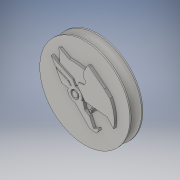
# Autodesk Inventor part: RTS Small Pharah Wheel
Saved by Autodesk Inventor 2016 (Build 200138000, 138)
## iProperties
Created: 2017-09-05
Part Number: RTS Small Pharah Wheel
Material: Generic
Document SubType Name: Modeling
Designer: Student
Density: 1 g/cm^3
Appearance: Default
Author: Student
Autodesk Inventor part; units mm, degrees
ref_plane "YZ Plane" through (0, 0, 0) normal (1, 0, 0) x (0, 1, 0)
ref_plane "XZ Plane" through (0, 0, 0) normal (0, 1, 0) x (-1, 0, 0)
ref_plane "XY Plane" through (0, 0, 0) normal (0, 0, 1) x (1, 0, 0)
sketch "Sketch1" plane through (0, 0, 0) normal (0, 0, 1) x (1, 0, 0)
  circle A0 centre (0, 0) radius 21.971
  dimension "d0" = 43.942
  constraints: 1 centre point, 1 coincident
  measures "d0" diameter of A0
extrude "Extrusion1" add sketch "Sketch1" along normal blind 6.35
sketch "Sketch3" plane through (0, 0, 0) normal (1, 0, 0) x (0, 1, 0)
  line L0 (21.971, 0) -> (21.971, 6.35) projected
  circle A0 centre (21.971, 3.175) radius 2.54
  line L1 (0, -1.27) -> (0, 7.62) projected
  point P0 (0, 0)
  dimension "d37" = 5.08
  constraints: 1 centre point, 1 midpoint
  measures "d37" diameter of A0
revolve "Revolution1" cut sketch "Sketch3" angle 360 about axis through (0, 0, -10) along (0, 0, 1)
sketch "Sketch4" plane through (0, 0, 0) normal (0, 0, -1) x (-1, 0, 0)
  line L0 (2.4384, -2.5883) -> (2.4384, 2.5883)
  line L1 (-2.4384, -2.5883) -> (-2.4384, 2.5883)
  arc A0 (2.4384, 2.5883) -> (-2.4384, 2.5883) centre (0, 0) ccw
  arc A1 (-2.4384, -2.5883) -> (2.4384, -2.5883) centre (0, 0) ccw
  dimension "d44" = 4.8768
  dimension "d45" = 3.556
  dimension "d46" = 5.1766
  dimension "d47" = 2.4384
  constraints: 4 end point, 4 point on circle, 2 centre point, 1 coincident, 1 parallel, 1 vertical
  measures "d44" distance between parallel lines of L1 L0
  measures "d45" radius of A0
  measures "d46" distance of L0.start L0.end
  measures "d47" distance from line of point (0, 0) L0
extrude "Extrusion3" cut sketch "Sketch4" against normal blind 5.2324
sketch "Sketch7" plane through (0, 0, 6.35) normal (0, 0, 1) x (1, 0, 0)
  line L0 (-16.6095, 17.2761) -> (16.9999, 17.2761) construction
  line L1 (16.9999, 17.2761) -> (16.9999, -16.3333) construction
  line L2 (16.9999, -16.3333) -> (-16.6095, -16.3333) construction
  line L3 (-16.6095, -16.3333) -> (-16.6095, 17.2761) construction
  line L4 (-11.6409, 13.9515) -> (-11.0896, 7.9216)
  line L5 (-10.846, 7.5655) -> (-4.1655, 4.5831)
  line L6 (-4.1655, 4.5831) -> (-3.2803, 2.7793)
  line L7 (-2.9643, 2.5005) -> (-2.215, 2.3615)
  arc A0 (-3.2803, 2.7793) -> (-2.9643, 2.5005) centre (-2.9521, 2.8328) ccw
  arc A1 (-11.0896, 7.9216) -> (-10.846, 7.5655) centre (-10.7308, 7.9057) ccw
  line L8 (-2.215, 2.3615) -> (-1.2053, 1.1357)
  circle A2 centre (-3.5155, -1.6738) radius 1.3912
  circle A3 centre (-3.5155, -1.6738) radius 1.9873
  arc A4 (-5.697, 1.0386) -> (-5.3458, 1.287) centre (-3.5155, -1.6738) ccw
  line L9 (-11.6409, 13.9515) -> (-10.9777, 13.9515)
  line L10 (-10.9777, 13.9515) -> (-6.6742, 11.6126)
  arc A5 (1.1675, 10.7462) -> (-6.6742, 11.6126) centre (-5.8633, -16.9682) ccw
  line L11 (1.1675, 10.7462) -> (2.608, 13.5351)
  arc A6 (3.3361, 13.55) -> (2.608, 13.5351) centre (2.9847, 12.9251) ccw
  line L12 (3.3361, 13.55) -> (10.8059, 7.7029)
  line L13 (10.8059, 7.7029) -> (13.5308, 5.0781)
  arc A7 (15.3657, -6.8873) -> (13.5308, 5.0781) centre (-3.032, -3.5852) ccw
  line L14 (15.3657, -6.8873) -> (12.1684, -3.357)
  line L15 (12.1684, -3.357) -> (7.5314, -2.8768)
  line L16 (7.5314, -2.8768) -> (7.0204, -3.2978)
  arc A8 (7.0204, -3.2978) -> (6.2865, -4.1165) centre (8.4411, -5.3095) ccw
  arc A9 (6.691, -2.8601) -> (6.2865, -4.1165) centre (9.098, -4.3284) ccw
  arc A10 (1.2675, -2.0364) -> (1.5721, -2.2799) centre (1.8757, -1.5881) ccw
  line L17 (1.2675, -2.0364) -> (-0.2802, -0.051)
  line L18 (-1.2053, 1.1357) -> (-0.2802, -0.051)
  line L19 (-15.1657, 8.8933) -> (-15.0771, 9.0065)
  line L20 (-15.0771, 9.0065) -> (-4.5214, 4.1672)
  line L21 (-4.5214, 4.1672) -> (-3.3907, 1.9212)
  line L22 (-6.652, 2.1979) -> (-5.6743, 1.0111)
  line L23 (-6.3027, 2.5826) -> (-5.3012, 1.2266)
  arc A11 (-5.6743, 1.0111) -> (-5.3012, 1.2266) centre (-5.5057, 1.15) ccw
  arc A12 (-6.652, 2.1979) -> (-7.0642, 2.431) centre (-7.2707, 1.5847) ccw
  arc A13 (-6.3027, 2.5826) -> (-6.6404, 2.7727) centre (-6.6833, 2.3015) ccw
  line L24 (-12.8802, 4.9767) -> (-7.0642, 2.431)
  line L25 (-6.6404, 2.7727) -> (-13.1518, 5.6227)
  line L26 (-13.1518, 5.6227) -> (-15.1657, 8.8933)
  line L27 (-12.8802, 4.9767) -> (-9.9722, -0.1277)
  line L28 (-9.9722, -0.1277) -> (-6.9287, -0.6545)
  arc A14 (4.2152, -5.0875) -> (3.7303, -4.5159) centre (3.6739, -5.0552) ccw
  arc A15 (3.7303, -4.5159) -> (3.0044, -5.147) centre (3.5903, -5.0878) ccw
  arc A16 (3.7824, -5.697) -> (4.2152, -5.0875) centre (3.5916, -5.1031) ccw
  arc A17 (3.2039, -5.3256) -> (3.7824, -5.697) centre (3.7454, -5.1184) ccw
  arc A18 (3.0044, -5.147) -> (3.7824, -6.3158) centre (4.0277, -5.3091) ccw
  arc A19 (3.1652, -5.3374) -> (3.7824, -6.0903) centre (3.8243, -5.4265) ccw
  arc A20 (3.2039, -5.3256) -> (3.1652, -5.3374) centre (3.1957, -5.3682) ccw
  arc A21 (3.7824, -6.0903) -> (4.3927, -5.66) centre (3.8814, -5.5828) ccw
  arc A22 (4.9875, -4.1165) -> (4.3927, -5.66) centre (12.9264, -8.0623) ccw
  arc A23 (3.7824, -6.3158) -> (4.654, -5.4642) centre (3.7228, -5.3829) ccw
  arc A24 (5.5077, -3.6657) -> (4.654, -5.4642) centre (11.7252, -7.7184) ccw
  line L29 (6.691, -2.8601) -> (6.7411, -2.781)
  line L30 (6.7411, -2.781) -> (6.2583, -2.745)
  arc A25 (6.2583, -2.745) -> (5.5077, -3.6657) centre (11.9972, -8.1901) ccw
  line L31 (1.5721, -2.2799) -> (6.0608, -2.7005)
  arc A26 (6.0608, -2.7005) -> (4.9875, -4.1165) centre (18.767, -13.4458) ccw
  line L32 (-6.9287, -0.6545) -> (-6.8497, -0.6741)
  line L33 (-3.4701, -5.1544) -> (3.5916, -12.454)
  line L34 (3.5916, -12.454) -> (6.7411, -12.9326)
  line L35 (6.7411, -12.9326) -> (8.2425, -11.189)
  line L36 (8.2425, -11.189) -> (7.7891, -10.5363)
  line L37 (7.7891, -10.5363) -> (6.1043, -11.3298)
  line L38 (6.1043, -11.3298) -> (5.7785, -11.4832)
  arc A27 (5.4757, -11.3297) -> (5.7785, -11.4832) centre (5.6869, -11.2886) ccw
  line L39 (5.4757, -11.3297) -> (3.5617, -7.266)
  line L40 (3.5617, -7.266) -> (1.2345, -5.8833)
  line L41 (1.2345, -5.8833) -> (0.3159, -2.4902)
  line L42 (0.3159, -2.4902) -> (-0.2289, -2.8205)
  line L43 (1.1675, 10.7462) -> (0.4371, 9.3321)
  line L44 (0.4371, 9.3321) -> (0.4371, 7.7029)
  line L45 (0.4371, 7.7029) -> (1.8757, 6.3431)
  line L46 (1.8757, 6.3431) -> (0.9998, 4.5316)
  line L47 (0.9998, 4.5316) -> (-1.3397, 4.3613)
  arc A28 (-1.3397, 4.3613) -> (-1.8021, 3.9921) centre (-1.3437, 3.8922) ccw
  line L48 (-1.8021, 3.9921) -> (-2.2406, 2.7138)
  arc A29 (-2.2406, 2.7138) -> (-2.215, 2.3615) centre (-2.0345, 2.5517) ccw
  line L49 (-3.3907, 1.9212) -> (-3.3394, 1.8026)
  line L50 (6.0608, -2.7005) -> (6.2583, -2.745)
  line L51 (6.7411, -2.781) -> (7.5314, -2.8768)
  point P0 (0, 0)
  constraints: 96 end point, 60 point on circle, 30 centre point, 3 tangent, 2 coincident, 2 point on line, 1 collinear, 1 horizontal, 1 parallel, 1 vertical, 2 other
extrude "Extrusion5" add sketch "Sketch7" along normal blind 1.016 contours L9 L10 A5 L43 L44 L45 L46 L47 A28 L48 A29 L7 A0 L6 L5 A1 L4 | L16 A8 A9 L29 L51 | L50 A25 A24 A23 A18 A15 A14 A16 A17 A20 A19 A21 A22 A26
extrude "Extrusion6" add sketch "Sketch7" along normal blind 1.27 contours L11 A6 L12 L13 A7 L14 L15 L51 L30 L50 L31 A10 L17 L18 L8 A29 L48 A28 L47 L46 L45 L44 L43 | A2 | L22 A11 L23 A4 | A4 L32 L28 L27 L24 A12 L22 | A4 L42 L41 L40 L39 A27 L38 L37 L36 L35 L34 L33 | L23 A13 L25 L26 L19 L20 L21 L49 A4
body "Solid1"
